Autodesk Inventor part; units mm, degrees
(part 2 of 4)
sketch "Кутник 125х14" plane through (0, 0, 0) normal (0, 0, 1) x (1, 0, 0)
  line L0 (-39.4035, -37.5892) -> (-39.4035, 87.4108)
  line L1 (-39.4035, 87.4108) -> (-30.0035, 87.4108)
  arc A0 (-25.4035, 82.8108) -> (-30.0035, 87.4108) centre (-30.0035, 82.8108) ccw
  line L2 (-25.4035, 82.8108) -> (-25.4035, -9.5892)
  arc A1 (-25.4035, -9.5892) -> (-11.4035, -23.5892) centre (-11.4035, -9.5892) ccw
  line L3 (-11.4035, -23.5892) -> (80.9965, -23.5892)
  arc A2 (85.5965, -28.1892) -> (80.9965, -23.5892) centre (80.9965, -28.1892) ccw
  line L4 (85.5965, -28.1892) -> (85.5965, -37.5892)
  line L5 (85.5965, -37.5892) -> (-39.4035, -37.5892)
  point P0 (8.2133, 8.2133)
  dimension "d276" = 125
  dimension "d277" = 14
  dimension "d278" = 14
  dimension "d279" = 4.6
  measures "d276" distance between parallel lines of L5 L1
  measures "d277" distance between parallel lines of L5 L3
  measures "d278" radius of A1
  measures "d279" radius of A2
sketch "Кутник 125х16" plane through (0, 0, 0) normal (0, 0, 1) x (1, 0, 0)
  line L0 (-40.4804, -38.5892) -> (-40.4804, 86.4108)
  line L1 (-40.4804, 86.4108) -> (-29.0804, 86.4108)
  arc A0 (-24.4804, 81.8108) -> (-29.0804, 86.4108) centre (-29.0804, 81.8108) ccw
  line L2 (-24.4804, 81.8108) -> (-24.4804, -8.5892)
  arc A1 (-24.4804, -8.5892) -> (-10.4804, -22.5892) centre (-10.4804, -8.5892) ccw
  line L3 (-10.4804, -22.5892) -> (79.9196, -22.5892)
  arc A2 (84.5196, -27.1892) -> (79.9196, -22.5892) centre (79.9196, -27.1892) ccw
  line L4 (84.5196, -27.1892) -> (84.5196, -38.5892)
  line L5 (84.5196, -38.5892) -> (-40.4804, -38.5892)
  point P0 (8.2133, 8.2133)
  dimension "d280" = 125
  dimension "d281" = 16
  dimension "d282" = 14
  dimension "d283" = 4.6
  measures "d280" distance between parallel lines of L5 L1
  measures "d281" distance between parallel lines of L5 L3
  measures "d282" radius of A1
  measures "d283" radius of A2
sketch "Кутник 140х9" plane through (0, 0, 0) normal (0, 0, 1) x (1, 0, 0)
  line L0 (-42.4804, -40.4464) -> (-42.4804, 99.5536)
  line L1 (-42.4804, 99.5536) -> (-38.0804, 99.5536)
  arc A0 (-33.4804, 94.9536) -> (-38.0804, 99.5536) centre (-38.0804, 94.9536) ccw
  line L2 (-33.4804, 94.9536) -> (-33.4804, -17.4464)
  arc A1 (-33.4804, -17.4464) -> (-19.4804, -31.4464) centre (-19.4804, -17.4464) ccw
  line L3 (-19.4804, -31.4464) -> (92.9196, -31.4464)
  arc A2 (97.5196, -36.0464) -> (92.9196, -31.4464) centre (92.9196, -36.0464) ccw
  line L4 (97.5196, -36.0464) -> (97.5196, -40.4464)
  line L5 (97.5196, -40.4464) -> (-42.4804, -40.4464)
  point P0 (8.2133, 8.2133)
  dimension "d284" = 140
  dimension "d285" = 9
  dimension "d286" = 14
  dimension "d287" = 4.6
  measures "d284" distance between parallel lines of L5 L1
  measures "d285" distance between parallel lines of L5 L3
  measures "d286" radius of A1
  measures "d287" radius of A2
sketch "Кутник 140х10" plane through (0, 0, 0) normal (0, 0, 1) x (1, 0, 0)
  line L0 (-43.0188, -40.9464) -> (-43.0188, 99.0536)
  line L1 (-43.0188, 99.0536) -> (-37.6188, 99.0536)
  arc A0 (-33.0188, 94.4536) -> (-37.6188, 99.0536) centre (-37.6188, 94.4536) ccw
  line L2 (-33.0188, 94.4536) -> (-33.0188, -16.9464)
  arc A1 (-33.0188, -16.9464) -> (-19.0188, -30.9464) centre (-19.0188, -16.9464) ccw
  line L3 (-19.0188, -30.9464) -> (92.3812, -30.9464)
  arc A2 (96.9812, -35.5464) -> (92.3812, -30.9464) centre (92.3812, -35.5464) ccw
  line L4 (96.9812, -35.5464) -> (96.9812, -40.9464)
  line L5 (96.9812, -40.9464) -> (-43.0188, -40.9464)
  point P0 (8.2133, 8.2133)
  dimension "d288" = 140
  dimension "d289" = 10
  dimension "d290" = 14
  dimension "d291" = 4.6
  measures "d288" distance between parallel lines of L5 L1
  measures "d289" distance between parallel lines of L5 L3
  measures "d290" radius of A1
  measures "d291" radius of A2
sketch "Кутник 140х12" plane through (0, 0, 0) normal (0, 0, 1) x (1, 0, 0)
  line L0 (-44.0958, -41.9464) -> (-44.0958, 98.0536)
  line L1 (-44.0958, 98.0536) -> (-36.6958, 98.0536)
  arc A0 (-32.0958, 93.4536) -> (-36.6958, 98.0536) centre (-36.6958, 93.4536) ccw
  line L2 (-32.0958, 93.4536) -> (-32.0958, -15.9464)
  arc A1 (-32.0958, -15.9464) -> (-18.0958, -29.9464) centre (-18.0958, -15.9464) ccw
  line L3 (-18.0958, -29.9464) -> (91.3042, -29.9464)
  arc A2 (95.9042, -34.5464) -> (91.3042, -29.9464) centre (91.3042, -34.5464) ccw
  line L4 (95.9042, -34.5464) -> (95.9042, -41.9464)
  line L5 (95.9042, -41.9464) -> (-44.0958, -41.9464)
  point P0 (8.2133, 8.2133)
  dimension "d292" = 140
  dimension "d293" = 12
  dimension "d294" = 14
  dimension "d295" = 4.6
  measures "d292" distance between parallel lines of L5 L1
  measures "d293" distance between parallel lines of L5 L3
  measures "d294" radius of A1
  measures "d295" radius of A2
sketch "Кутник 160х10" plane through (0, 0, 0) normal (0, 0, 1) x (1, 0, 0)
  line L0 (-50.8035, -48.175) -> (-50.8035, 111.825)
  line L1 (-50.8035, 111.825) -> (-46.1035, 111.825)
  arc A0 (-40.8035, 106.525) -> (-46.1035, 111.825) centre (-46.1035, 106.525) ccw
  line L2 (-40.8035, 106.525) -> (-40.8035, -22.175)
  arc A1 (-40.8035, -22.175) -> (-24.8035, -38.175) centre (-24.8035, -22.175) ccw
  line L3 (-24.8035, -38.175) -> (103.8965, -38.175)
  arc A2 (109.1965, -43.475) -> (103.8965, -38.175) centre (103.8965, -43.475) ccw
  line L4 (109.1965, -43.475) -> (109.1965, -48.175)
  line L5 (109.1965, -48.175) -> (-50.8035, -48.175)
  point P0 (8.2133, 8.2133)
  dimension "d296" = 160
  dimension "d297" = 10
  dimension "d298" = 16
  dimension "d299" = 5.3
  measures "d296" distance between parallel lines of L5 L1
  measures "d297" distance between parallel lines of L5 L3
  measures "d298" radius of A1
  measures "d299" radius of A2
sketch "Кутник 160х11" plane through (0, 0, 0) normal (0, 0, 1) x (1, 0, 0)
  line L0 (-51.3419, -48.675) -> (-51.3419, 111.325)
  line L1 (-51.3419, 111.325) -> (-45.6419, 111.325)
  arc A0 (-40.3419, 106.025) -> (-45.6419, 111.325) centre (-45.6419, 106.025) ccw
  line L2 (-40.3419, 106.025) -> (-40.3419, -21.675)
  arc A1 (-40.3419, -21.675) -> (-24.3419, -37.675) centre (-24.3419, -21.675) ccw
  line L3 (-24.3419, -37.675) -> (103.3581, -37.675)
  arc A2 (108.6581, -42.975) -> (103.3581, -37.675) centre (103.3581, -42.975) ccw
  line L4 (108.6581, -42.975) -> (108.6581, -48.675)
  line L5 (108.6581, -48.675) -> (-51.3419, -48.675)
  point P0 (8.2133, 8.2133)
  dimension "d12" = 25
  dimension "d13" = 4
  dimension "d14" = 3.5
  dimension "d15" = 1.2
  dimension "d56" = 45
  dimension "d57" = 5
  dimension "d58" = 5
  dimension "d59" = 1.7
  dimension "d300" = 160
  dimension "d301" = 11
  dimension "d302" = 16
  dimension "d303" = 5.3
  measures "d300" distance between parallel lines of L5 L1
  measures "d301" distance between parallel lines of L5 L3
  measures "d302" radius of A1
  measures "d303" radius of A2
sketch "Кутник 160х12" plane through (0, 0, 0) normal (0, 0, 1) x (1, 0, 0)
  line L0 (-51.8804, -49.175) -> (-51.8804, 110.825)
  line L1 (-51.8804, 110.825) -> (-45.1804, 110.825)
  arc A0 (-39.8804, 105.525) -> (-45.1804, 110.825) centre (-45.1804, 105.525) ccw
  line L2 (-39.8804, 105.525) -> (-39.8804, -21.175)
  arc A1 (-39.8804, -21.175) -> (-23.8804, -37.175) centre (-23.8804, -21.175) ccw
  line L3 (-23.8804, -37.175) -> (102.8196, -37.175)
  arc A2 (108.1196, -42.475) -> (102.8196, -37.175) centre (102.8196, -42.475) ccw
  line L4 (108.1196, -42.475) -> (108.1196, -49.175)
  line L5 (108.1196, -49.175) -> (-51.8804, -49.175)
  point P0 (8.2133, 8.2133)
  dimension "d304" = 160
  dimension "d305" = 12
  dimension "d306" = 16
  dimension "d307" = 5.3
  measures "d304" distance between parallel lines of L5 L1
  measures "d305" distance between parallel lines of L5 L3
  measures "d306" radius of A1
  measures "d307" radius of A2
sketch "Кутник 160х14" plane through (0, 0, 0) normal (0, 0, 1) x (1, 0, 0)
  line L0 (-52.9573, -50.175) -> (-52.9573, 109.825)
  line L1 (-52.9573, 109.825) -> (-44.2573, 109.825)
  arc A0 (-38.9573, 104.525) -> (-44.2573, 109.825) centre (-44.2573, 104.525) ccw
  line L2 (-38.9573, 104.525) -> (-38.9573, -20.175)
  arc A1 (-38.9573, -20.175) -> (-22.9573, -36.175) centre (-22.9573, -20.175) ccw
  line L3 (-22.9573, -36.175) -> (101.7427, -36.175)
  arc A2 (107.0427, -41.475) -> (101.7427, -36.175) centre (101.7427, -41.475) ccw
  line L4 (107.0427, -41.475) -> (107.0427, -50.175)
  line L5 (107.0427, -50.175) -> (-52.9573, -50.175)
  point P0 (8.2133, 8.2133)
  dimension "d308" = 160
  dimension "d309" = 14
  dimension "d310" = 16
  dimension "d311" = 5.3
  measures "d308" distance between parallel lines of L5 L1
  measures "d309" distance between parallel lines of L5 L3
  measures "d310" radius of A1
  measures "d311" radius of A2
sketch "Кутник 160х16" plane through (0, 0, 0) normal (0, 0, 1) x (1, 0, 0)
  line L0 (-54.0342, -51.175) -> (-54.0342, 108.825)
  line L1 (-54.0342, 108.825) -> (-43.3342, 108.825)
  arc A0 (-38.0342, 103.525) -> (-43.3342, 108.825) centre (-43.3342, 103.525) ccw
  line L2 (-38.0342, 103.525) -> (-38.0342, -19.175)
  arc A1 (-38.0342, -19.175) -> (-22.0342, -35.175) centre (-22.0342, -19.175) ccw
  line L3 (-22.0342, -35.175) -> (100.6658, -35.175)
  arc A2 (105.9658, -40.475) -> (100.6658, -35.175) centre (100.6658, -40.475) ccw
  line L4 (105.9658, -40.475) -> (105.9658, -51.175)
  line L5 (105.9658, -51.175) -> (-54.0342, -51.175)
  point P0 (8.2133, 8.2133)
  dimension "d312" = 160
  dimension "d313" = 16
  dimension "d314" = 16
  dimension "d315" = 5.3
  measures "d312" distance between parallel lines of L5 L1
  measures "d313" distance between parallel lines of L5 L3
  measures "d314" radius of A1
  measures "d315" radius of A2
sketch "Кутник 160х18" plane through (0, 0, 0) normal (0, 0, 1) x (1, 0, 0)
  line L0 (-55.1112, -52.175) -> (-55.1112, 107.825)
  line L1 (-55.1112, 107.825) -> (-42.4112, 107.825)
  arc A0 (-37.1112, 102.525) -> (-42.4112, 107.825) centre (-42.4112, 102.525) ccw
  line L2 (-37.1112, 102.525) -> (-37.1112, -18.175)
  arc A1 (-37.1112, -18.175) -> (-21.1112, -34.175) centre (-21.1112, -18.175) ccw
  line L3 (-21.1112, -34.175) -> (99.5888, -34.175)
  arc A2 (104.8888, -39.475) -> (99.5888, -34.175) centre (99.5888, -39.475) ccw
  line L4 (104.8888, -39.475) -> (104.8888, -52.175)
  line L5 (104.8888, -52.175) -> (-55.1112, -52.175)
  point P0 (8.2133, 8.2133)
  dimension "d316" = 160
  dimension "d317" = 18
  dimension "d318" = 16
  dimension "d319" = 5.3
  measures "d316" distance between parallel lines of L5 L1
  measures "d317" distance between parallel lines of L5 L3
  measures "d318" radius of A1
  measures "d319" radius of A2
sketch "Кутник 160х20" plane through (0, 0, 0) normal (0, 0, 1) x (1, 0, 0)
  line L0 (-56.1881, -53.175) -> (-56.1881, 106.825)
  line L1 (-56.1881, 106.825) -> (-41.4881, 106.825)
  arc A0 (-36.1881, 101.525) -> (-41.4881, 106.825) centre (-41.4881, 101.525) ccw
  line L2 (-36.1881, 101.525) -> (-36.1881, -17.175)
  arc A1 (-36.1881, -17.175) -> (-20.1881, -33.175) centre (-20.1881, -17.175) ccw
  line L3 (-20.1881, -33.175) -> (98.5119, -33.175)
  arc A2 (103.8119, -38.475) -> (98.5119, -33.175) centre (98.5119, -38.475) ccw
  line L4 (103.8119, -38.475) -> (103.8119, -53.175)
  line L5 (103.8119, -53.175) -> (-56.1881, -53.175)
  point P0 (8.2133, 8.2133)
  dimension "d320" = 160
  dimension "d321" = 20
  dimension "d322" = 16
  dimension "d323" = 5.3
  measures "d320" distance between parallel lines of L5 L1
  measures "d321" distance between parallel lines of L5 L3
  measures "d322" radius of A1
  measures "d323" radius of A2
sketch "Кутник 180х11" plane through (0, 0, 0) normal (0, 0, 1) x (1, 0, 0)
  line L0 (-59.0342, -55.8178) -> (-59.0342, 124.1822)
  line L1 (-59.0342, 124.1822) -> (-53.3342, 124.1822)
  arc A0 (-48.0342, 118.8822) -> (-53.3342, 124.1822) centre (-53.3342, 118.8822) ccw
  line L2 (-48.0342, 118.8822) -> (-48.0342, -28.8178)
  arc A1 (-48.0342, -28.8178) -> (-32.0342, -44.8178) centre (-32.0342, -28.8178) ccw
  line L3 (-32.0342, -44.8178) -> (115.6658, -44.8178)
  arc A2 (120.9658, -50.1178) -> (115.6658, -44.8178) centre (115.6658, -50.1178) ccw
  line L4 (120.9658, -50.1178) -> (120.9658, -55.8178)
  line L5 (120.9658, -55.8178) -> (-59.0342, -55.8178)
  point P0 (8.2133, 8.2133)
  dimension "d324" = 180
  dimension "d325" = 11
  dimension "d326" = 16
  dimension "d327" = 5.3
  measures "d324" distance between parallel lines of L5 L1
  measures "d325" distance between parallel lines of L5 L3
  measures "d326" radius of A1
  measures "d327" radius of A2
sketch "Кутник 180х12" plane through (0, 0, 0) normal (0, 0, 1) x (1, 0, 0)
  line L0 (-59.5727, -56.3178) -> (-59.5727, 123.6822)
  line L1 (-59.5727, 123.6822) -> (-52.8727, 123.6822)
  arc A0 (-47.5727, 118.3822) -> (-52.8727, 123.6822) centre (-52.8727, 118.3822) ccw
  line L2 (-47.5727, 118.3822) -> (-47.5727, -28.3178)
  arc A1 (-47.5727, -28.3178) -> (-31.5727, -44.3178) centre (-31.5727, -28.3178) ccw
  line L3 (-31.5727, -44.3178) -> (115.1273, -44.3178)
  arc A2 (120.4273, -49.6178) -> (115.1273, -44.3178) centre (115.1273, -49.6178) ccw
  line L4 (120.4273, -49.6178) -> (120.4273, -56.3178)
  line L5 (120.4273, -56.3178) -> (-59.5727, -56.3178)
  point P0 (8.2133, 8.2133)
  dimension "d328" = 180
  dimension "d329" = 12
  dimension "d330" = 16
  dimension "d331" = 5.3
  measures "d328" distance between parallel lines of L5 L1
  measures "d329" distance between parallel lines of L5 L3
  measures "d330" radius of A1
  measures "d331" radius of A2
sketch "Кутник 200х12" plane through (0, 0, 0) normal (0, 0, 1) x (1, 0, 0)
  line L0 (-67.3573, -63.5464) -> (-67.3573, 136.4536)
  line L1 (-67.3573, 136.4536) -> (-61.3573, 136.4536)
  arc A0 (-55.3573, 130.4536) -> (-61.3573, 136.4536) centre (-61.3573, 130.4536) ccw
  line L2 (-55.3573, 130.4536) -> (-55.3573, -33.5464)
  arc A1 (-55.3573, -33.5464) -> (-37.3573, -51.5464) centre (-37.3573, -33.5464) ccw
  line L3 (-37.3573, -51.5464) -> (126.6427, -51.5464)
  arc A2 (132.6427, -57.5464) -> (126.6427, -51.5464) centre (126.6427, -57.5464) ccw
  line L4 (132.6427, -57.5464) -> (132.6427, -63.5464)
  line L5 (132.6427, -63.5464) -> (-67.3573, -63.5464)
  point P0 (8.2133, 8.2133)
  dimension "d332" = 200
  dimension "d333" = 12
  dimension "d334" = 18
  dimension "d335" = 6
  measures "d332" distance between parallel lines of L5 L1
  measures "d333" distance between parallel lines of L5 L3
  measures "d334" radius of A1
  measures "d335" radius of A2
sketch "Кутник 200х13" plane through (0, 0, 0) normal (0, 0, 1) x (1, 0, 0)
  line L0 (-67.8958, -64.0464) -> (-67.8958, 135.9536)
  line L1 (-67.8958, 135.9536) -> (-60.8958, 135.9536)
  arc A0 (-54.8958, 129.9536) -> (-60.8958, 135.9536) centre (-60.8958, 129.9536) ccw
  line L2 (-54.8958, 129.9536) -> (-54.8958, -33.0464)
  arc A1 (-54.8958, -33.0464) -> (-36.8958, -51.0464) centre (-36.8958, -33.0464) ccw
  line L3 (-36.8958, -51.0464) -> (126.1042, -51.0464)
  arc A2 (132.1042, -57.0464) -> (126.1042, -51.0464) centre (126.1042, -57.0464) ccw
  line L4 (132.1042, -57.0464) -> (132.1042, -64.0464)
  line L5 (132.1042, -64.0464) -> (-67.8958, -64.0464)
  point P0 (8.2133, 8.2133)
  dimension "d336" = 200
  dimension "d337" = 13
  dimension "d338" = 18
  dimension "d339" = 6
  measures "d336" distance between parallel lines of L5 L1
  measures "d337" distance between parallel lines of L5 L3
  measures "d338" radius of A1
  measures "d339" radius of A2
sketch "Кутник 200х14" plane through (0, 0, 0) normal (0, 0, 1) x (1, 0, 0)
  line L0 (-68.4342, -64.5464) -> (-68.4342, 135.4536)
  line L1 (-68.4342, 135.4536) -> (-60.4342, 135.4536)
  arc A0 (-54.4342, 129.4536) -> (-60.4342, 135.4536) centre (-60.4342, 129.4536) ccw
  line L2 (-54.4342, 129.4536) -> (-54.4342, -32.5464)
  arc A1 (-54.4342, -32.5464) -> (-36.4342, -50.5464) centre (-36.4342, -32.5464) ccw
  line L3 (-36.4342, -50.5464) -> (125.5658, -50.5464)
  arc A2 (131.5658, -56.5464) -> (125.5658, -50.5464) centre (125.5658, -56.5464) ccw
  line L4 (131.5658, -56.5464) -> (131.5658, -64.5464)
  line L5 (131.5658, -64.5464) -> (-68.4342, -64.5464)
  point P0 (8.2133, 8.2133)
  dimension "d340" = 200
  dimension "d341" = 14
  dimension "d342" = 18
  dimension "d343" = 6
  measures "d340" distance between parallel lines of L5 L1
  measures "d341" distance between parallel lines of L5 L3
  measures "d342" radius of A1
  measures "d343" radius of A2
sketch "Кутник 200х16" plane through (0, 0, 0) normal (0, 0, 1) x (1, 0, 0)
  line L0 (-69.5112, -65.5464) -> (-69.5112, 134.4536)
  line L1 (-69.5112, 134.4536) -> (-59.5112, 134.4536)
  arc A0 (-53.5112, 128.4536) -> (-59.5112, 134.4536) centre (-59.5112, 128.4536) ccw
  line L2 (-53.5112, 128.4536) -> (-53.5112, -31.5464)
  arc A1 (-53.5112, -31.5464) -> (-35.5112, -49.5464) centre (-35.5112, -31.5464) ccw
  line L3 (-35.5112, -49.5464) -> (124.4888, -49.5464)
  arc A2 (130.4888, -55.5464) -> (124.4888, -49.5464) centre (124.4888, -55.5464) ccw
  line L4 (130.4888, -55.5464) -> (130.4888, -65.5464)
  line L5 (130.4888, -65.5464) -> (-69.5112, -65.5464)
  point P0 (8.2133, 8.2133)
  dimension "d344" = 200
  dimension "d345" = 16
  dimension "d346" = 18
  dimension "d347" = 6
  measures "d344" distance between parallel lines of L5 L1
  measures "d345" distance between parallel lines of L5 L3
  measures "d346" radius of A1
  measures "d347" radius of A2
sketch "Кутник 200х20" plane through (0, 0, 0) normal (0, 0, 1) x (1, 0, 0)
  line L0 (-71.665, -67.5464) -> (-71.665, 132.4536)
  line L1 (-71.665, 132.4536) -> (-57.665, 132.4536)
  arc A0 (-51.665, 126.4536) -> (-57.665, 132.4536) centre (-57.665, 126.4536) ccw
  line L2 (-51.665, 126.4536) -> (-51.665, -29.5464)
  arc A1 (-51.665, -29.5464) -> (-33.665, -47.5464) centre (-33.665, -29.5464) ccw
  line L3 (-33.665, -47.5464) -> (122.335, -47.5464)
  arc A2 (128.335, -53.5464) -> (122.335, -47.5464) centre (122.335, -53.5464) ccw
  line L4 (128.335, -53.5464) -> (128.335, -67.5464)
  line L5 (128.335, -67.5464) -> (-71.665, -67.5464)
  point P0 (8.2133, 8.2133)
  dimension "d348" = 200
  dimension "d349" = 20
  dimension "d350" = 18
  dimension "d351" = 6
  measures "d348" distance between parallel lines of L5 L1
  measures "d349" distance between parallel lines of L5 L3
  measures "d350" radius of A1
  measures "d351" radius of A2
sketch "Кутник 200х25" plane through (0, 0, 0) normal (0, 0, 1) x (1, 0, 0)
  line L0 (-74.3573, -70.0464) -> (-74.3573, 129.9536)
  line L1 (-74.3573, 129.9536) -> (-55.3573, 129.9536)
  arc A0 (-49.3573, 123.9536) -> (-55.3573, 129.9536) centre (-55.3573, 123.9536) ccw
  line L2 (-49.3573, 123.9536) -> (-49.3573, -27.0464)
  arc A1 (-49.3573, -27.0464) -> (-31.3573, -45.0464) centre (-31.3573, -27.0464) ccw
  line L3 (-31.3573, -45.0464) -> (119.6427, -45.0464)
  arc A2 (125.6427, -51.0464) -> (119.6427, -45.0464) centre (119.6427, -51.0464) ccw
  line L4 (125.6427, -51.0464) -> (125.6427, -70.0464)
  line L5 (125.6427, -70.0464) -> (-74.3573, -70.0464)
  point P0 (8.2133, 8.2133)
  dimension "d352" = 200
  dimension "d353" = 25
  dimension "d354" = 18
  dimension "d355" = 6
  measures "d352" distance between parallel lines of L5 L1
  measures "d353" distance between parallel lines of L5 L3
  measures "d354" radius of A1
  measures "d355" radius of A2
sketch "Кутник 200х30" plane through (0, 0, 0) normal (0, 0, 1) x (1, 0, 0)
  line L0 (-77.0496, -72.5464) -> (-77.0496, 127.4536)
  line L1 (-77.0496, 127.4536) -> (-53.0496, 127.4536)
  arc A0 (-47.0496, 121.4536) -> (-53.0496, 127.4536) centre (-53.0496, 121.4536) ccw
  line L2 (-47.0496, 121.4536) -> (-47.0496, -24.5464)
  arc A1 (-47.0496, -24.5464) -> (-29.0496, -42.5464) centre (-29.0496, -24.5464) ccw
  line L3 (-29.0496, -42.5464) -> (116.9504, -42.5464)
  arc A2 (122.9504, -48.5464) -> (116.9504, -42.5464) centre (116.9504, -48.5464) ccw
  line L4 (122.9504, -48.5464) -> (122.9504, -72.5464)
  line L5 (122.9504, -72.5464) -> (-77.0496, -72.5464)
  point P0 (8.2133, 8.2133)
  dimension "d356" = 200
  dimension "d357" = 30
  dimension "d358" = 18
  dimension "d359" = 6
  measures "d356" distance between parallel lines of L5 L1
  measures "d357" distance between parallel lines of L5 L3
  measures "d358" radius of A1
  measures "d359" radius of A2
sketch "Кутник 220х14" plane through (0, 0, 0) normal (0, 0, 1) x (1, 0, 0)
  line L0 (-76.2804, -71.8321) -> (-76.2804, 148.1679)
  line L1 (-76.2804, 148.1679) -> (-69.2804, 148.1679)
  arc A0 (-62.2804, 141.1679) -> (-69.2804, 148.1679) centre (-69.2804, 141.1679) ccw
  line L2 (-62.2804, 141.1679) -> (-62.2804, -36.8321)
  arc A1 (-62.2804, -36.8321) -> (-41.2804, -57.8321) centre (-41.2804, -36.8321) ccw
  line L3 (-41.2804, -57.8321) -> (136.7196, -57.8321)
  arc A2 (143.7196, -64.8321) -> (136.7196, -57.8321) centre (136.7196, -64.8321) ccw
  line L4 (143.7196, -64.8321) -> (143.7196, -71.8321)
  line L5 (143.7196, -71.8321) -> (-76.2804, -71.8321)
  point P0 (8.2133, 8.2133)
  dimension "d360" = 220
  dimension "d361" = 14
  dimension "d362" = 21
  dimension "d363" = 7
  measures "d360" distance between parallel lines of L5 L1
  measures "d361" distance between parallel lines of L5 L3
  measures "d362" radius of A1
  measures "d363" radius of A2
sketch "Кутник 220х16" plane through (0, 0, 0) normal (0, 0, 1) x (1, 0, 0)
  line L0 (-77.3573, -72.8321) -> (-77.3573, 147.1679)
  line L1 (-77.3573, 147.1679) -> (-68.3573, 147.1679)
  arc A0 (-61.3573, 140.1679) -> (-68.3573, 147.1679) centre (-68.3573, 140.1679) ccw
  line L2 (-61.3573, 140.1679) -> (-61.3573, -35.8321)
  arc A1 (-61.3573, -35.8321) -> (-40.3573, -56.8321) centre (-40.3573, -35.8321) ccw
  line L3 (-40.3573, -56.8321) -> (135.6427, -56.8321)
  arc A2 (142.6427, -63.8321) -> (135.6427, -56.8321) centre (135.6427, -63.8321) ccw
  line L4 (142.6427, -63.8321) -> (142.6427, -72.8321)
  line L5 (142.6427, -72.8321) -> (-77.3573, -72.8321)
  point P0 (8.2133, 8.2133)
  dimension "d368" = 220
  dimension "d369" = 16
  dimension "d370" = 21
  dimension "d371" = 7
  measures "d368" distance between parallel lines of L5 L1
  measures "d369" distance between parallel lines of L5 L3
  measures "d370" radius of A1
  measures "d371" radius of A2
sketch "Кутник 250х16" plane through (0, 0, 0) normal (0, 0, 1) x (1, 0, 0)
  line L0 (-89.0496, -83.6892) -> (-89.0496, 166.3108)
  line L1 (-89.0496, 166.3108) -> (-81.0496, 166.3108)
  arc A0 (-73.0496, 158.3108) -> (-81.0496, 166.3108) centre (-81.0496, 158.3108) ccw
  line L2 (-73.0496, 158.3108) -> (-73.0496, -43.6892)
  arc A1 (-73.0496, -43.6892) -> (-49.0496, -67.6892) centre (-49.0496, -43.6892) ccw
  line L3 (-49.0496, -67.6892) -> (152.9504, -67.6892)
  arc A2 (160.9504, -75.6892) -> (152.9504, -67.6892) centre (152.9504, -75.6892) ccw
  line L4 (160.9504, -75.6892) -> (160.9504, -83.6892)
  line L5 (160.9504, -83.6892) -> (-89.0496, -83.6892)
  point P0 (8.2133, 8.2133)
  dimension "d372" = 250
  dimension "d373" = 16
  dimension "d374" = 24
  dimension "d375" = 8
  measures "d372" distance between parallel lines of L5 L1
  measures "d373" distance between parallel lines of L5 L3
  measures "d374" radius of A1
  measures "d375" radius of A2
sketch "Кутник 250х18" plane through (0, 0, 0) normal (0, 0, 1) x (1, 0, 0)
  line L0 (-90.1265, -84.6892) -> (-90.1265, 165.3108)
  line L1 (-90.1265, 165.3108) -> (-80.1265, 165.3108)
  arc A0 (-72.1265, 157.3108) -> (-80.1265, 165.3108) centre (-80.1265, 157.3108) ccw
  line L2 (-72.1265, 157.3108) -> (-72.1265, -42.6892)
  arc A1 (-72.1265, -42.6892) -> (-48.1265, -66.6892) centre (-48.1265, -42.6892) ccw
  line L3 (-48.1265, -66.6892) -> (151.8735, -66.6892)
  arc A2 (159.8735, -74.6892) -> (151.8735, -66.6892) centre (151.8735, -74.6892) ccw
  line L4 (159.8735, -74.6892) -> (159.8735, -84.6892)
  line L5 (159.8735, -84.6892) -> (-90.1265, -84.6892)
  point P0 (8.2133, 8.2133)
  dimension "d376" = 250
  dimension "d377" = 18
  dimension "d378" = 24
  dimension "d379" = 8
  measures "d376" distance between parallel lines of L5 L1
  measures "d377" distance between parallel lines of L5 L3
  measures "d378" radius of A1
  measures "d379" radius of A2
sketch "Кутник 250х20" plane through (0, 0, 0) normal (0, 0, 1) x (1, 0, 0)
  line L0 (-91.2035, -85.6892) -> (-91.2035, 164.3108)
  line L1 (-91.2035, 164.3108) -> (-79.2035, 164.3108)
  arc A0 (-71.2035, 156.3108) -> (-79.2035, 164.3108) centre (-79.2035, 156.3108) ccw
  line L2 (-71.2035, 156.3108) -> (-71.2035, -41.6892)
  arc A1 (-71.2035, -41.6892) -> (-47.2035, -65.6892) centre (-47.2035, -41.6892) ccw
  line L3 (-47.2035, -65.6892) -> (150.7965, -65.6892)
  arc A2 (158.7965, -73.6892) -> (150.7965, -65.6892) centre (150.7965, -73.6892) ccw
  line L4 (158.7965, -73.6892) -> (158.7965, -85.6892)
  line L5 (158.7965, -85.6892) -> (-91.2035, -85.6892)
  point P0 (8.2133, 8.2133)
  dimension "d380" = 250
  dimension "d381" = 20
  dimension "d382" = 24
  dimension "d383" = 8
  measures "d380" distance between parallel lines of L5 L1
  measures "d381" distance between parallel lines of L5 L3
  measures "d382" radius of A1
  measures "d383" radius of A2
sketch "Кутник 250х22" plane through (0, 0, 0) normal (0, 0, 1) x (1, 0, 0)
  line L0 (-92.2804, -86.6892) -> (-92.2804, 163.3108)
  line L1 (-92.2804, 163.3108) -> (-78.2804, 163.3108)
  arc A0 (-70.2804, 155.3108) -> (-78.2804, 163.3108) centre (-78.2804, 155.3108) ccw
  line L2 (-70.2804, 155.3108) -> (-70.2804, -40.6892)
  arc A1 (-70.2804, -40.6892) -> (-46.2804, -64.6892) centre (-46.2804, -40.6892) ccw
  line L3 (-46.2804, -64.6892) -> (149.7196, -64.6892)
  arc A2 (157.7196, -72.6892) -> (149.7196, -64.6892) centre (149.7196, -72.6892) ccw
  line L4 (157.7196, -72.6892) -> (157.7196, -86.6892)
  line L5 (157.7196, -86.6892) -> (-92.2804, -86.6892)
  point P0 (8.2133, 8.2133)
  dimension "d384" = 250
  dimension "d385" = 22
  dimension "d386" = 24
  dimension "d387" = 8
  measures "d384" distance between parallel lines of L5 L1
  measures "d385" distance between parallel lines of L5 L3
  measures "d386" radius of A1
  measures "d387" radius of A2
sketch "Кутник 250х25" plane through (0, 0, 0) normal (0, 0, 1) x (1, 0, 0)
  line L0 (-93.8958, -88.1892) -> (-93.8958, 161.8108)
  line L1 (-93.8958, 161.8108) -> (-76.8958, 161.8108)
  arc A0 (-68.8958, 153.8108) -> (-76.8958, 161.8108) centre (-76.8958, 153.8108) ccw
  line L2 (-68.8958, 153.8108) -> (-68.8958, -39.1892)
  arc A1 (-68.8958, -39.1892) -> (-44.8958, -63.1892) centre (-44.8958, -39.1892) ccw
  line L3 (-44.8958, -63.1892) -> (148.1042, -63.1892)
  arc A2 (156.1042, -71.1892) -> (148.1042, -63.1892) centre (148.1042, -71.1892) ccw
  line L4 (156.1042, -71.1892) -> (156.1042, -88.1892)
  line L5 (156.1042, -88.1892) -> (-93.8958, -88.1892)
  point P0 (8.2133, 8.2133)
  dimension "d388" = 250
  dimension "d389" = 25
  dimension "d390" = 24
  dimension "d391" = 8
  measures "d388" distance between parallel lines of L5 L1
  measures "d389" distance between parallel lines of L5 L3
  measures "d390" radius of A1
  measures "d391" radius of A2
sketch "Кутник 250х28" plane through (0, 0, 0) normal (0, 0, 1) x (1, 0, 0)
  line L0 (-95.5112, -89.6892) -> (-95.5112, 160.3108)
  line L1 (-95.5112, 160.3108) -> (-75.5112, 160.3108)
  arc A0 (-67.5112, 152.3108) -> (-75.5112, 160.3108) centre (-75.5112, 152.3108) ccw
  line L2 (-67.5112, 152.3108) -> (-67.5112, -37.6892)
  arc A1 (-67.5112, -37.6892) -> (-43.5112, -61.6892) centre (-43.5112, -37.6892) ccw
  line L3 (-43.5112, -61.6892) -> (146.4888, -61.6892)
  arc A2 (154.4888, -69.6892) -> (146.4888, -61.6892) centre (146.4888, -69.6892) ccw
  line L4 (154.4888, -69.6892) -> (154.4888, -89.6892)
  line L5 (154.4888, -89.6892) -> (-95.5112, -89.6892)
  point P0 (8.2133, 8.2133)
  dimension "d392" = 250
  dimension "d393" = 28
  dimension "d394" = 24
  dimension "d395" = 8
  measures "d392" distance between parallel lines of L5 L1
  measures "d393" distance between parallel lines of L5 L3
  measures "d394" radius of A1
  measures "d395" radius of A2
sketch "Кутник 250х30" plane through (0, 0, 0) normal (0, 0, 1) x (1, 0, 0)
  line L0 (-96.5881, -90.6892) -> (-96.5881, 159.3108)
  line L1 (-96.5881, 159.3108) -> (-74.5881, 159.3108)
  arc A0 (-66.5881, 151.3108) -> (-74.5881, 159.3108) centre (-74.5881, 151.3108) ccw
  line L2 (-66.5881, 151.3108) -> (-66.5881, -36.6892)
  arc A1 (-66.5881, -36.6892) -> (-42.5881, -60.6892) centre (-42.5881, -36.6892) ccw
  line L3 (-42.5881, -60.6892) -> (145.4119, -60.6892)
  arc A2 (153.4119, -68.6892) -> (145.4119, -60.6892) centre (145.4119, -68.6892) ccw
  line L4 (153.4119, -68.6892) -> (153.4119, -90.6892)
  line L5 (153.4119, -90.6892) -> (-96.5881, -90.6892)
  point P0 (8.2133, 8.2133)
  dimension "d396" = 250
  dimension "d397" = 30
  dimension "d398" = 24
  dimension "d399" = 8
  measures "d396" distance between parallel lines of L5 L1
  measures "d397" distance between parallel lines of L5 L3
  measures "d398" radius of A1
  measures "d399" radius of A2
sketch "Швелер 5" plane through (0, 0, 0) normal (0, 0, 1) x (1, 0, 0)
  line L0 (27.0973, 56.2463) -> (27.0973, 32.2463)
  line L1 (54.6973, 19.2463) -> (22.6973, 19.2463)
  line L2 (22.6973, 19.2463) -> (22.6973, 69.2463)
  line L3 (22.6973, 69.2463) -> (54.6973, 69.2463)
  line L4 (52.1973, 62.2463) -> (33.0973, 62.2463)
  arc A0 (33.0973, 62.2463) -> (27.0973, 56.2463) centre (33.0973, 56.2463) ccw
  arc A1 (27.0973, 32.2463) -> (33.0973, 26.2463) centre (33.0973, 32.2463) ccw
  line L5 (33.0973, 26.2463) -> (52.1973, 26.2463)
  line L6 (54.6973, 19.2463) -> (54.6973, 23.7463)
  arc A2 (54.6973, 23.7463) -> (52.1973, 26.2463) centre (52.1973, 23.7463) ccw
  line L7 (54.6973, 69.2463) -> (54.6973, 64.7463)
  arc A3 (52.1973, 62.2463) -> (54.6973, 64.7463) centre (52.1973, 64.7463) ccw
  point P0 (39.2152, 43.3464)
  dimension "d404" = 32
  dimension "d405" = 50
  dimension "d406" = 4.4
  dimension "d407" = 6
  dimension "d408" = 2.5
  dimension "d409" = 7
  dimension "d410" = 2.5
  measures "d404" distance of L1.start L1.end
  measures "d405" distance of L1.end L2.end
  measures "d406" distance between parallel lines of L2 L0
  measures "d407" radius of A1
  measures "d408" radius of A2
  measures "d409" distance between parallel lines of L1 L5
  measures "d410" radius of A3
sketch "Швелер 6.5" plane through (0, 0, 0) normal (0, 0, 1) x (1, 0, 0)
  line L0 (24.9796, 63.5463) -> (24.9796, 24.9463)
  line L1 (56.5796, 11.7463) -> (20.5796, 11.7463)
  line L2 (20.5796, 11.7463) -> (20.5796, 76.7463)
  line L3 (20.5796, 76.7463) -> (56.5796, 76.7463)
  line L4 (54.0796, 69.5463) -> (30.9796, 69.5463)
  arc A0 (30.9796, 69.5463) -> (24.9796, 63.5463) centre (30.9796, 63.5463) ccw
  arc A1 (24.9796, 24.9463) -> (30.9796, 18.9463) centre (30.9796, 24.9463) ccw
  line L5 (30.9796, 18.9463) -> (54.0796, 18.9463)
  line L6 (56.5796, 11.7463) -> (56.5796, 16.4463)
  arc A2 (56.5796, 16.4463) -> (54.0796, 18.9463) centre (54.0796, 16.4463) ccw
  line L7 (56.5796, 76.7463) -> (56.5796, 72.0463)
  arc A3 (54.0796, 69.5463) -> (56.5796, 72.0463) centre (54.0796, 72.0463) ccw
  point P0 (39.2152, 43.3464)
  dimension "d411" = 36
  dimension "d412" = 65
  dimension "d413" = 4.4
  dimension "d414" = 6
  dimension "d415" = 2.5
  dimension "d416" = 7.2
  measures "d411" distance of L1.start L1.end
  measures "d412" distance of L1.end L2.end
  measures "d413" distance between parallel lines of L2 L0
  measures "d414" radius of A1
  measures "d415" radius of A2
  measures "d416" distance between parallel lines of L1 L5
sketch "Швелер 8" plane through (0, 0, 0) normal (0, 0, 1) x (1, 0, 0)
  line L0 (22.8149, 70.3463) -> (22.8149, 18.1463)
  line L1 (58.3149, 4.2463) -> (18.3149, 4.2463)
  line L2 (18.3149, 4.2463) -> (18.3149, 84.2463)
  line L3 (18.3149, 84.2463) -> (58.3149, 84.2463)
  line L4 (55.8149, 76.8463) -> (29.3149, 76.8463)
  arc A0 (29.3149, 76.8463) -> (22.8149, 70.3463) centre (29.3149, 70.3463) ccw
  arc A1 (22.8149, 18.1463) -> (29.3149, 11.6463) centre (29.3149, 18.1463) ccw
  line L5 (29.3149, 11.6463) -> (55.8149, 11.6463)
  line L6 (58.3149, 4.2463) -> (58.3149, 9.1463)
  arc A2 (58.3149, 9.1463) -> (55.8149, 11.6463) centre (55.8149, 9.1463) ccw
  line L7 (58.3149, 84.2463) -> (58.3149, 79.3463)
  arc A3 (55.8149, 76.8463) -> (58.3149, 79.3463) centre (55.8149, 79.3463) ccw
  point P0 (39.2152, 43.3464)
  dimension "d417" = 40
  dimension "d418" = 80
  dimension "d419" = 4.5
  dimension "d420" = 6.5
  dimension "d421" = 2.5
  dimension "d422" = 7.4
  measures "d417" distance of L1.start L1.end
  measures "d418" distance of L1.end L2.end
  measures "d419" distance between parallel lines of L2 L0
  measures "d420" radius of A1
  measures "d421" radius of A2
  measures "d422" distance between parallel lines of L1 L5
sketch "Швелер 10" plane through (0, 0, 0) normal (0, 0, 1) x (1, 0, 0)
  line L0 (19.6384, 79.6463) -> (19.6384, 8.8463)
  line L1 (61.1384, -5.7537) -> (15.1384, -5.7537)
  line L2 (15.1384, -5.7537) -> (15.1384, 94.2463)
  line L3 (15.1384, 94.2463) -> (61.1384, 94.2463)
  line L4 (58.1384, 86.6463) -> (26.6384, 86.6463)
  arc A0 (26.6384, 86.6463) -> (19.6384, 79.6463) centre (26.6384, 79.6463) ccw
  arc A1 (19.6384, 8.8463) -> (26.6384, 1.8463) centre (26.6384, 8.8463) ccw
  line L5 (26.6384, 1.8463) -> (58.1384, 1.8463)
  line L6 (61.1384, -5.7537) -> (61.1384, -1.1537)
  arc A2 (61.1384, -1.1537) -> (58.1384, 1.8463) centre (58.1384, -1.1537) ccw
  line L7 (61.1384, 94.2463) -> (61.1384, 89.6463)
  arc A3 (58.1384, 86.6463) -> (61.1384, 89.6463) centre (58.1384, 89.6463) ccw
  point P0 (39.2152, 43.3464)
  dimension "d423" = 46
  dimension "d424" = 100
  dimension "d425" = 4.5
  dimension "d426" = 7
  dimension "d427" = 3
  dimension "d428" = 7.6
  measures "d423" distance of L1.start L1.end
  measures "d424" distance of L1.end L2.end
  measures "d425" distance between parallel lines of L2 L0
  measures "d426" radius of A1
  measures "d427" radius of A2
  measures "d428" distance between parallel lines of L1 L5
sketch "Швелер 12" plane through (0, 0, 0) normal (0, 0, 1) x (1, 0, 0)
  line L0 (16.5561, 88.9463) -> (16.5561, -0.4537)
  line L1 (63.7561, -15.7537) -> (11.7561, -15.7537)
  line L2 (11.7561, -15.7537) -> (11.7561, 104.2463)
  line L3 (11.7561, 104.2463) -> (63.7561, 104.2463)
  line L4 (60.7561, 96.4463) -> (24.0561, 96.4463)
  arc A0 (24.0561, 96.4463) -> (16.5561, 88.9463) centre (24.0561, 88.9463) ccw
  arc A1 (16.5561, -0.4537) -> (24.0561, -7.9537) centre (24.0561, -0.4537) ccw
  line L5 (24.0561, -7.9537) -> (60.7561, -7.9537)
  line L6 (63.7561, -15.7537) -> (63.7561, -10.9537)
  arc A2 (63.7561, -10.9537) -> (60.7561, -7.9537) centre (60.7561, -10.9537) ccw
  line L7 (63.7561, 104.2463) -> (63.7561, 99.4463)
  arc A3 (60.7561, 96.4463) -> (63.7561, 99.4463) centre (60.7561, 99.4463) ccw
  point P0 (39.2152, 43.3464)
  dimension "d326" = 16
  dimension "d429" = 52
  dimension "d430" = 120
  dimension "d431" = 4.8
  dimension "d432" = 7.5
  dimension "d433" = 3
  dimension "d434" = 7.8
  measures "d429" distance of L1.start L1.end
  measures "d430" distance of L1.end L2.end
  measures "d431" distance between parallel lines of L2 L0
  measures "d432" radius of A1
  measures "d433" radius of A2
  measures "d434" distance between parallel lines of L1 L5
sketch "Швелер 14" plane through (0, 0, 0) normal (0, 0, 1) x (1, 0, 0)
  line L0 (13.3326, 98.1463) -> (13.3326, -9.6537)
  line L1 (66.4326, -25.7537) -> (8.4326, -25.7537)
  line L2 (8.4326, -25.7537) -> (8.4326, 114.2463)
  line L3 (8.4326, 114.2463) -> (66.4326, 114.2463)
  line L4 (63.4326, 106.1463) -> (21.3326, 106.1463)
  arc A0 (21.3326, 106.1463) -> (13.3326, 98.1463) centre (21.3326, 98.1463) ccw
  arc A1 (13.3326, -9.6537) -> (21.3326, -17.6537) centre (21.3326, -9.6537) ccw
  line L5 (21.3326, -17.6537) -> (63.4326, -17.6537)
  line L6 (66.4326, -25.7537) -> (66.4326, -20.6537)
  arc A2 (66.4326, -20.6537) -> (63.4326, -17.6537) centre (63.4326, -20.6537) ccw
  line L7 (66.4326, 114.2463) -> (66.4326, 109.1463)
  arc A3 (63.4326, 106.1463) -> (66.4326, 109.1463) centre (63.4326, 109.1463) ccw
  point P0 (39.2152, 43.3464)
  dimension "d435" = 58
  dimension "d436" = 140
  dimension "d437" = 4.9
  dimension "d438" = 8
  dimension "d439" = 3
  dimension "d440" = 8.1
  measures "d435" distance of L1.start L1.end
  measures "d436" distance of L1.end L2.end
  measures "d437" distance between parallel lines of L2 L0
  measures "d438" radius of A1
  measures "d439" radius of A2
  measures "d440" distance between parallel lines of L1 L5
sketch "Швелер 14а" plane through (0, 0, 0) normal (0, 0, 1) x (1, 0, 0)
  line L0 (11.2149, 97.5463) -> (11.2149, -9.0537)
  line L1 (68.3149, -25.7537) -> (6.3149, -25.7537)
  line L2 (6.3149, -25.7537) -> (6.3149, 114.2463)
  line L3 (6.3149, 114.2463) -> (68.3149, 114.2463)
  line L4 (65.3149, 105.5463) -> (19.2149, 105.5463)
  arc A0 (19.2149, 105.5463) -> (11.2149, 97.5463) centre (19.2149, 97.5463) ccw
  arc A1 (11.2149, -9.0537) -> (19.2149, -17.0537) centre (19.2149, -9.0537) ccw
  line L5 (19.2149, -17.0537) -> (65.3149, -17.0537)
  line L6 (68.3149, -25.7537) -> (68.3149, -20.0537)
  arc A2 (68.3149, -20.0537) -> (65.3149, -17.0537) centre (65.3149, -20.0537) ccw
  line L7 (68.3149, 114.2463) -> (68.3149, 108.5463)
  arc A3 (65.3149, 105.5463) -> (68.3149, 108.5463) centre (65.3149, 108.5463) ccw
  point P0 (39.2152, 43.3464)
  dimension "d441" = 62
  dimension "d442" = 140
  dimension "d443" = 4.9
  dimension "d444" = 8
  dimension "d445" = 3
  dimension "d446" = 8.7
  measures "d441" distance of L1.start L1.end
  measures "d442" distance of L1.end L2.end
  measures "d443" distance between parallel lines of L2 L0
  measures "d444" radius of A1
  measures "d445" radius of A2
  measures "d446" distance between parallel lines of L1 L5
sketch "Швелер 16" plane through (0, 0, 0) normal (0, 0, 1) x (1, 0, 0)
  line L0 (10.2267, 107.3463) -> (10.2267, -18.8537)
  line L1 (69.2267, -35.7537) -> (5.2267, -35.7537)
  line L2 (5.2267, -35.7537) -> (5.2267, 124.2463)
  line L3 (5.2267, 124.2463) -> (69.2267, 124.2463)
  line L4 (65.7267, 115.8463) -> (18.7267, 115.8463)
  arc A0 (18.7267, 115.8463) -> (10.2267, 107.3463) centre (18.7267, 107.3463) ccw
  arc A1 (10.2267, -18.8537) -> (18.7267, -27.3537) centre (18.7267, -18.8537) ccw
  line L5 (18.7267, -27.3537) -> (65.7267, -27.3537)
  line L6 (69.2267, -35.7537) -> (69.2267, -30.8537)
  arc A2 (69.2267, -30.8537) -> (65.7267, -27.3537) centre (65.7267, -30.8537) ccw
  line L7 (69.2267, 124.2463) -> (69.2267, 119.3463)
  arc A3 (65.7267, 115.8463) -> (69.2267, 119.3463) centre (65.7267, 119.3463) ccw
  point P0 (39.2152, 43.3464)
  dimension "d447" = 64
  dimension "d448" = 160
  dimension "d449" = 5
  dimension "d450" = 8.5
  dimension "d451" = 3.5
  dimension "d452" = 8.4
  measures "d447" distance of L1.start L1.end
  measures "d448" distance of L1.end L2.end
  measures "d449" distance between parallel lines of L2 L0
  measures "d450" radius of A1
  measures "d451" radius of A2
  measures "d452" distance between parallel lines of L1 L5
sketch "Швелер 16а" plane through (0, 0, 0) normal (0, 0, 1) x (1, 0, 0)
  line L0 (8.109, 106.7463) -> (8.109, -18.2537)
  line L1 (71.109, -35.7537) -> (3.109, -35.7537)
  line L2 (3.109, -35.7537) -> (3.109, 124.2463)
  line L3 (3.109, 124.2463) -> (71.109, 124.2463)
  line L4 (67.609, 115.2463) -> (16.609, 115.2463)
  arc A0 (16.609, 115.2463) -> (8.109, 106.7463) centre (16.609, 106.7463) ccw
  arc A1 (8.109, -18.2537) -> (16.609, -26.7537) centre (16.609, -18.2537) ccw
  line L5 (16.609, -26.7537) -> (67.609, -26.7537)
  line L6 (71.109, -35.7537) -> (71.109, -30.2537)
  arc A2 (71.109, -30.2537) -> (67.609, -26.7537) centre (67.609, -30.2537) ccw
  line L7 (71.109, 124.2463) -> (71.109, 118.7463)
  arc A3 (67.609, 115.2463) -> (71.109, 118.7463) centre (67.609, 118.7463) ccw
  point P0 (39.2152, 43.3464)
  dimension "d453" = 68
  dimension "d454" = 160
  dimension "d455" = 5
  dimension "d456" = 8.5
  dimension "d457" = 3.5
  dimension "d458" = 9
  measures "d453" distance of L1.start L1.end
  measures "d454" distance of L1.end L2.end
  measures "d455" distance between parallel lines of L2 L0
  measures "d456" radius of A1
  measures "d457" radius of A2
  measures "d458" distance between parallel lines of L1 L5
sketch "Швелер 18" plane through (0, 0, 0) normal (0, 0, 1) x (1, 0, 0)
  line L0 (7.0031, 116.5463) -> (7.0031, -28.0537)
  line L1 (71.9031, -45.7537) -> (1.9031, -45.7537)
  line L2 (1.9031, -45.7537) -> (1.9031, 134.2463)
  line L3 (1.9031, 134.2463) -> (71.9031, 134.2463)
  line L4 (68.4031, 125.5463) -> (16.0031, 125.5463)
  arc A0 (16.0031, 125.5463) -> (7.0031, 116.5463) centre (16.0031, 116.5463) ccw
  arc A1 (7.0031, -28.0537) -> (16.0031, -37.0537) centre (16.0031, -28.0537) ccw
  line L5 (16.0031, -37.0537) -> (68.4031, -37.0537)
  line L6 (71.9031, -45.7537) -> (71.9031, -40.5537)
  arc A2 (71.9031, -40.5537) -> (68.4031, -37.0537) centre (68.4031, -40.5537) ccw
  line L7 (71.9031, 134.2463) -> (71.9031, 129.0463)
  arc A3 (68.4031, 125.5463) -> (71.9031, 129.0463) centre (68.4031, 129.0463) ccw
  point P0 (39.2152, 43.3464)
  dimension "d459" = 70
  dimension "d460" = 180
  dimension "d461" = 5.1
  dimension "d462" = 9
  dimension "d463" = 3.5
  dimension "d464" = 8.7
  measures "d459" distance of L1.start L1.end
  measures "d460" distance of L1.end L2.end
  measures "d461" distance between parallel lines of L2 L0
  measures "d462" radius of A1
  measures "d463" radius of A2
  measures "d464" distance between parallel lines of L1 L5
sketch "Швелер 18а" plane through (0, 0, 0) normal (0, 0, 1) x (1, 0, 0)
  line L0 (4.8855, 115.9463) -> (4.8855, -27.4537)
  line L1 (73.7855, -45.7537) -> (-0.2145, -45.7537)
  line L2 (-0.2145, -45.7537) -> (-0.2145, 134.2463)
  line L3 (-0.2145, 134.2463) -> (73.7855, 134.2463)
  line L4 (70.2855, 124.9463) -> (13.8855, 124.9463)
  arc A0 (13.8855, 124.9463) -> (4.8855, 115.9463) centre (13.8855, 115.9463) ccw
  arc A1 (4.8855, -27.4537) -> (13.8855, -36.4537) centre (13.8855, -27.4537) ccw
  line L5 (13.8855, -36.4537) -> (70.2855, -36.4537)
  line L6 (73.7855, -45.7537) -> (73.7855, -39.9537)
  arc A2 (73.7855, -39.9537) -> (70.2855, -36.4537) centre (70.2855, -39.9537) ccw
  line L7 (73.7855, 134.2463) -> (73.7855, 128.4463)
  arc A3 (70.2855, 124.9463) -> (73.7855, 128.4463) centre (70.2855, 128.4463) ccw
  point P0 (39.2152, 43.3464)
  dimension "d465" = 74
  dimension "d466" = 180
  dimension "d467" = 5.1
  dimension "d468" = 9
  dimension "d469" = 3.5
  dimension "d470" = 9.3
  measures "d465" distance of L1.start L1.end
  measures "d466" distance of L1.end L2.end
  measures "d467" distance between parallel lines of L2 L0
  measures "d468" radius of A1
  measures "d469" radius of A2
  measures "d470" distance between parallel lines of L1 L5
sketch "Швелер 20" plane through (0, 0, 0) normal (0, 0, 1) x (1, 0, 0)
  line L0 (3.8973, 125.7463) -> (3.8973, -37.2537)
  line L1 (74.6973, -55.7537) -> (-1.3027, -55.7537)
  line L2 (-1.3027, -55.7537) -> (-1.3027, 144.2463)
  line L3 (-1.3027, 144.2463) -> (74.6973, 144.2463)
  line L4 (70.6973, 135.2463) -> (13.3973, 135.2463)
  arc A0 (13.3973, 135.2463) -> (3.8973, 125.7463) centre (13.3973, 125.7463) ccw
  arc A1 (3.8973, -37.2537) -> (13.3973, -46.7537) centre (13.3973, -37.2537) ccw
  line L5 (13.3973, -46.7537) -> (70.6973, -46.7537)
  line L6 (74.6973, -55.7537) -> (74.6973, -50.7537)
  arc A2 (74.6973, -50.7537) -> (70.6973, -46.7537) centre (70.6973, -50.7537) ccw
  line L7 (74.6973, 144.2463) -> (74.6973, 139.2463)
  arc A3 (70.6973, 135.2463) -> (74.6973, 139.2463) centre (70.6973, 139.2463) ccw
  point P0 (39.2152, 43.3464)
  dimension "d471" = 76
  dimension "d472" = 200
  dimension "d473" = 5.2
  dimension "d474" = 9.5
  dimension "d475" = 4
  dimension "d476" = 9
  measures "d471" distance of L1.start L1.end
  measures "d472" distance of L1.end L2.end
  measures "d473" distance between parallel lines of L2 L0
  measures "d474" radius of A1
  measures "d475" radius of A2
  measures "d476" distance between parallel lines of L1 L5
sketch "Швелер 20а" plane through (0, 0, 0) normal (0, 0, 1) x (1, 0, 0)
  line L0 (1.7796, 125.0463) -> (1.7796, -36.5537)
  line L1 (76.5796, -55.7537) -> (-3.4204, -55.7537)
  line L2 (-3.4204, -55.7537) -> (-3.4204, 144.2463)
  line L3 (-3.4204, 144.2463) -> (76.5796, 144.2463)
  line L4 (72.5796, 134.5463) -> (11.2796, 134.5463)
  arc A0 (11.2796, 134.5463) -> (1.7796, 125.0463) centre (11.2796, 125.0463) ccw
  arc A1 (1.7796, -36.5537) -> (11.2796, -46.0537) centre (11.2796, -36.5537) ccw
  line L5 (11.2796, -46.0537) -> (72.5796, -46.0537)
  line L6 (76.5796, -55.7537) -> (76.5796, -50.0537)
  arc A2 (76.5796, -50.0537) -> (72.5796, -46.0537) centre (72.5796, -50.0537) ccw
  line L7 (76.5796, 144.2463) -> (76.5796, 138.5463)
  arc A3 (72.5796, 134.5463) -> (76.5796, 138.5463) centre (72.5796, 138.5463) ccw
  point P0 (39.2152, 43.3464)
  dimension "d477" = 80
  dimension "d478" = 200
  dimension "d479" = 5.2
  dimension "d480" = 9.5
  dimension "d481" = 4
  dimension "d482" = 9.7
  measures "d477" distance of L1.start L1.end
  measures "d478" distance of L1.end L2.end
  measures "d479" distance between parallel lines of L2 L0
  measures "d480" radius of A1
  measures "d481" radius of A2
  measures "d482" distance between parallel lines of L1 L5
sketch "Швелер 22" plane through (0, 0, 0) normal (0, 0, 1) x (1, 0, 0)
  line L0 (0.7443, 134.7463) -> (0.7443, -46.2537)
  line L1 (77.3443, -65.7537) -> (-4.6557, -65.7537)
  line L2 (-4.6557, -65.7537) -> (-4.6557, 154.2463)
  line L3 (-4.6557, 154.2463) -> (77.3443, 154.2463)
  line L4 (73.3443, 144.7463) -> (10.7443, 144.7463)
  arc A0 (10.7443, 144.7463) -> (0.7443, 134.7463) centre (10.7443, 134.7463) ccw
  arc A1 (0.7443, -46.2537) -> (10.7443, -56.2537) centre (10.7443, -46.2537) ccw
  line L5 (10.7443, -56.2537) -> (73.3443, -56.2537)
  line L6 (77.3443, -65.7537) -> (77.3443, -60.2537)
  arc A2 (77.3443, -60.2537) -> (73.3443, -56.2537) centre (73.3443, -60.2537) ccw
  line L7 (77.3443, 154.2463) -> (77.3443, 148.7463)
  arc A3 (73.3443, 144.7463) -> (77.3443, 148.7463) centre (73.3443, 148.7463) ccw
  point P0 (39.2152, 43.3464)
  dimension "d483" = 82
  dimension "d484" = 220
  dimension "d485" = 5.4
  dimension "d486" = 10
  dimension "d487" = 4
  dimension "d488" = 9.5
  measures "d483" distance of L1.start L1.end
  measures "d484" distance of L1.end L2.end
  measures "d485" distance between parallel lines of L2 L0
  measures "d486" radius of A1
  measures "d487" radius of A2
  measures "d488" distance between parallel lines of L1 L5
sketch "Швелер 22а" plane through (0, 0, 0) normal (0, 0, 1) x (1, 0, 0)
  line L0 (-1.9027, 133.7463) -> (-1.9027, -45.2537)
  line L1 (79.6973, -65.7537) -> (-7.3027, -65.7537)
  line L2 (-7.3027, -65.7537) -> (-7.3027, 154.2463)
  line L3 (-7.3027, 154.2463) -> (79.6973, 154.2463)
  line L4 (75.6973, 143.7463) -> (8.0973, 143.7463)
  arc A0 (8.0973, 143.7463) -> (-1.9027, 133.7463) centre (8.0973, 133.7463) ccw
  arc A1 (-1.9027, -45.2537) -> (8.0973, -55.2537) centre (8.0973, -45.2537) ccw
  line L5 (8.0973, -55.2537) -> (75.6973, -55.2537)
  line L6 (79.6973, -65.7537) -> (79.6973, -59.2537)
  arc A2 (79.6973, -59.2537) -> (75.6973, -55.2537) centre (75.6973, -59.2537) ccw
  line L7 (79.6973, 154.2463) -> (79.6973, 147.7463)
  arc A3 (75.6973, 143.7463) -> (79.6973, 147.7463) centre (75.6973, 147.7463) ccw
  point P0 (39.2152, 43.3464)
  dimension "d489" = 87
  dimension "d490" = 220
  dimension "d491" = 5.4
  dimension "d492" = 10
  dimension "d493" = 4
  dimension "d494" = 10.5
  measures "d489" distance of L1.start L1.end
  measures "d490" distance of L1.end L2.end
  measures "d491" distance between parallel lines of L2 L0
  measures "d492" radius of A1
  measures "d493" radius of A2
  measures "d494" distance between parallel lines of L1 L5
sketch "Швелер 24" plane through (0, 0, 0) normal (0, 0, 1) x (1, 0, 0)
  line L0 (-3.4674, 143.7463) -> (-3.4674, -55.2537)
  line L1 (80.9326, -75.7537) -> (-9.0674, -75.7537)
  line L2 (-9.0674, -75.7537) -> (-9.0674, 164.2463)
  line L3 (-9.0674, 164.2463) -> (80.9326, 164.2463)
  line L4 (76.9326, 154.2463) -> (7.0326, 154.2463)
  arc A0 (7.0326, 154.2463) -> (-3.4674, 143.7463) centre (7.0326, 143.7463) ccw
  arc A1 (-3.4674, -55.2537) -> (7.0326, -65.7537) centre (7.0326, -55.2537) ccw
  line L5 (7.0326, -65.7537) -> (76.9326, -65.7537)
  line L6 (80.9326, -75.7537) -> (80.9326, -69.7537)
  arc A2 (80.9326, -69.7537) -> (76.9326, -65.7537) centre (76.9326, -69.7537) ccw
  line L7 (80.9326, 164.2463) -> (80.9326, 158.2463)
  arc A3 (76.9326, 154.2463) -> (80.9326, 158.2463) centre (76.9326, 158.2463) ccw
  point P0 (39.2152, 43.3464)
  dimension "d495" = 90
  dimension "d496" = 240
  dimension "d497" = 5.6
  dimension "d498" = 10.5
  dimension "d499" = 4
  dimension "d500" = 10
  measures "d495" distance of L1.start L1.end
  measures "d496" distance of L1.end L2.end
  measures "d497" distance between parallel lines of L2 L0
  measures "d498" radius of A1
  measures "d499" radius of A2
  measures "d500" distance between parallel lines of L1 L5